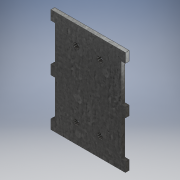
# Autodesk Inventor part: CAR BOTTOM PLATE
Saved by Autodesk Inventor 2017 (Build 210142000, 142)
## iProperties
Part Number: CAR BOTTOM PLATE
Material: Genérico
Document SubType Name: Modeling
Designer: Cristian
Density: 1 g/cm^3
Appearance: Valor por defecto
Author: Cristian
Autodesk Inventor part; units mm, degrees
ref_plane "YZ Plane" through (0, 0, 0) normal (1, 0, 0) x (0, 1, 0)
ref_plane "XZ Plane" through (0, 0, 0) normal (0, 1, 0) x (-1, 0, 0)
ref_plane "XY Plane" through (0, 0, 0) normal (0, 0, 1) x (1, 0, 0)
sketch "Boceto1" plane through (0, 0, 0) normal (0, 1, 0) x (-1, 0, 0)
  line L0 (0, 0) -> (88.9, 0)
  line L1 (88.9, 0) -> (88.9, -139.7)
  line L2 (88.9, -139.7) -> (0, -139.7)
  line L3 (0, -139.7) -> (0, 0)
  circle A0 centre (60.325, -25.4) radius 3.9688
  circle A1 centre (60.325, -114.3) radius 3.9688
  circle A2 centre (28.575, -25.4) radius 3.9687
  circle A3 centre (28.575, -114.3) radius 3.9687
  line L4 (88.9, 0) -> (94.4562, 0)
  line L5 (94.4562, 0) -> (94.4562, -12.7)
  line L6 (94.4562, -12.7) -> (88.9, -12.7)
  line L7 (88.9, -12.7) -> (88.9, 0)
  line L8 (88.9, -139.7) -> (94.4563, -139.7)
  line L9 (94.4563, -139.7) -> (94.4563, -127)
  line L10 (94.4563, -127) -> (88.9, -127)
  line L11 (88.9, -127) -> (88.9, -139.7)
  line L12 (0, 0) -> (-5.5563, 0)
  line L13 (-5.5563, 0) -> (-5.5563, -12.7)
  line L14 (-5.5563, -12.7) -> (0, -12.7)
  line L15 (0, -12.7) -> (0, 0)
  line L16 (0, -139.7) -> (-5.5562, -139.7)
  line L17 (-5.5562, -139.7) -> (-5.5562, -127)
  line L18 (-5.5562, -127) -> (0, -127)
  line L19 (0, -127) -> (0, -139.7)
  line L20 (88.9, -63.5) -> (94.4562, -63.5)
  line L21 (94.4562, -63.5) -> (94.4562, -76.2)
  line L22 (94.4562, -76.2) -> (88.9, -76.2)
  line L23 (88.9, -76.2) -> (88.9, -63.5)
  line L24 (0, -63.5) -> (-5.5563, -63.5)
  line L25 (-5.5563, -63.5) -> (-5.5563, -76.2)
  line L26 (-5.5563, -76.2) -> (0, -76.2)
  line L27 (0, -76.2) -> (0, -63.5)
  dimension "d0" = 88.9
  dimension "d1" = 139.7
  dimension "d2" = 7.9375
  dimension "d3" = 7.9375
  dimension "d4" = 7.9375
  dimension "d5" = 7.9375
  dimension "d6" = 88.9
  dimension "d7" = 28.575
  dimension "d8" = 28.575
  dimension "d9" = 28.575
  dimension "d10" = 28.575
  dimension "d11" = 25.4
  dimension "d12" = 25.4
  dimension "d13" = 88.9
  dimension "d17" = 5.5563
  dimension "d18" = 12.7
  dimension "d19" = 5.5563
  dimension "d20" = 12.7
  dimension "d21" = 5.5563
  dimension "d22" = 12.7
  dimension "d23" = 5.5563
  dimension "d24" = 12.7
  dimension "d25" = 5.5563
  dimension "d26" = 12.7
  dimension "d27" = 5.5563
  dimension "d28" = 12.7
  dimension "d29" = 63.5
  dimension "d30" = 63.5
  constraints: 56 end point, 14 parallel, 7 horizontal, 7 perpendicular, 4 centre point, 2 point on line
  measures "d0" distance between parallel lines of L3 L1
  measures "d1" distance of L0.end L1.end
  measures "d2" diameter of A0
  measures "d3" diameter of A1
  measures "d4" diameter of A2
  measures "d5" diameter of A3
  measures "d6" distance of A1.centre A0.centre
  measures "d7" distance from line of L3 A2.centre
  measures "d8" distance from line of L3 A3.centre
  measures "d9" distance from line of L1 A0.centre
  measures "d10" distance from line of L1 A1.centre
  measures "d11" distance from line of L0 A0.centre
  measures "d12" distance from line of L0 A2.centre
  measures "d13" distance of A2.centre A3.centre
  measures "d17" distance of L5.end L6.end
  measures "d18" distance of L4.end L5.end
  measures "d19" distance of L10.end L9.end
  measures "d20" distance of L9.end L8.end
  measures "d21" distance of L14.end L13.end
  measures "d22" distance of L13.end L12.end
  measures "d23" distance of L17.end L18.end
  measures "d24" distance of L16.end L17.end
  measures "d25" distance of L21.end L22.end
  measures "d26" distance of L20.end L21.end
  measures "d27" distance of L26.end L25.end
  measures "d28" distance of L25.end L24.end
  measures "d29" distance between parallel lines of L24 L12
  measures "d30" distance between parallel lines of L20 L4
extrude "Extrusión1" add sketch "Boceto1" along normal blind 5
